# Autodesk Inventor part: JUMPER3
Saved by Autodesk Inventor 2015 SP1 (Build 190203100, 203)
## iProperties
Created: 2015-06-25
Part Number: JUMPER3
Material: Generic
Document SubType Name: Modeling
Designer: Patrick
Density: 1 g/cm^3
Appearance: JUMPER3, JUMPER3
Author: Patrick
Autodesk Inventor part; units mm, degrees
ref_plane "YZ Plane" through (0, 0, 0) normal (1, 0, 0) x (0, 1, 0)
ref_plane "XZ Plane" through (0, 0, 0) normal (0, 1, 0) x (-1, 0, 0)
ref_plane "XY Plane" through (0, 0, 0) normal (0, 0, 1) x (1, 0, 0)
sketch "JUMPER3, JUMPER3_180" plane through (0, 0, 0) normal (0, 0, 1) x (1, 0, 0)
  line L0 (-1.395, -3.935) -> (-1.395, 3.935)
  line L1 (-1.395, 3.935) -> (1.395, 3.935)
  line L2 (1.395, 3.935) -> (1.395, -3.935)
  line L3 (1.395, -3.935) -> (-1.395, -3.935)
  constraints: 8 end point
extrude "Extrusion1" add sketch "JUMPER3, JUMPER3_180" along normal blind 1
body "Solid1"
